Autodesk Inventor part; units mm, degrees
(part 2 of 3)
  arc A210 (-114.4847, -238.4545) -> (-108.2711, -237.6145) centre (-111.4451, -237.537) ccw projected
  arc A211 (-82.9809, -239.5618) -> (-81.2537, -236.3199) centre (-93.2079, -232.032) ccw projected
  arc A212 (-79.039, -235.4413) -> (-81.2537, -236.3199) centre (-79.7594, -236.8559) ccw projected
  line L73 (-79.039, -235.4413) -> (-73.2785, -238.3744) projected
  arc A213 (-72.5842, -240.5094) -> (-73.2785, -238.3744) centre (-73.9989, -239.7891) ccw projected
  line L74 (-72.5842, -240.5094) -> (-73.4026, -242.1166) projected
  arc A214 (-82.2866, -251.3886) -> (-73.4026, -242.1166) centre (-93.2079, -232.032) ccw projected
  arc A215 (-86.1924, -246.4835) -> (-82.2866, -251.3886) centre (-83.8468, -248.6233) ccw projected
  arc A216 (-86.1924, -246.4835) -> (-82.9809, -239.5618) centre (-95.5749, -237.9244) ccw projected
  line L75 (-36.7385, 25.1704) -> (-35.059, 27.3253) projected
  arc A217 (-31.1029, 31.7555) -> (-35.059, 27.3253) centre (0, 0) ccw projected
  arc A218 (-25.7245, 29.1468) -> (-31.1029, 31.7555) centre (-28.8812, 29.4873) ccw projected
  arc A219 (-25.7245, 29.1468) -> (-25.6629, 24.5535) centre (-6.7844, 27.1038) ccw projected
  arc A220 (-28.6757, 20.9563) -> (-25.6629, 24.5535) centre (-28.8093, 24.1285) ccw projected
  arc A221 (-28.6757, 20.9563) -> (-33.3257, 20.1764) centre (-27.8737, 1.9232) ccw projected
  arc A222 (-36.7385, 25.1704) -> (-33.3257, 20.1764) centre (-34.2343, 23.2186) ccw projected
  arc A223 (35.5169, -0.0989) -> (38.7459, 3.1685) centre (23.6807, 14.8279) ccw projected
  arc A224 (44.4304, 1.3195) -> (38.7459, 3.1685) centre (41.2568, 1.2252) ccw projected
  arc A225 (43.8282, -7.409) -> (44.4304, 1.3195) centre (0, 0) ccw projected
  arc A226 (37.9436, -8.4597) -> (43.8282, -7.409) centre (40.6976, -6.8798) ccw projected
  arc A227 (37.9436, -8.4597) -> (35.1939, -4.7799) centre (21.4199, -17.9397) ccw projected
  arc A228 (35.5169, -0.0989) -> (35.1939, -4.7799) centre (37.4896, -2.5866) ccw projected
  arc A229 (11.0693, 33.748) -> (8.9598, 37.8287) centre (-6.7844, 27.1038) ccw projected
  arc A230 (12.4749, 42.6636) -> (8.9598, 37.8287) centre (11.5838, 39.6162) ccw projected
  arc A231 (20.59, 39.3936) -> (12.4749, 42.6636) centre (0, 0) ccw projected
  arc A232 (19.7709, 33.4723) -> (20.59, 39.3936) centre (19.1193, 36.5798) ccw projected
  arc A233 (19.7709, 33.4723) -> (15.4215, 31.9943) centre (23.6807, 14.8279) ccw projected
  arc A234 (11.0693, 33.748) -> (15.4215, 31.9943) centre (14.045, 34.8554) ccw projected
  point P0 (0, 0)
  point P1 (-30.4878, -157.8365)
  point P2 (-86.8989, -84.1298)
  point P3 (-18.5783, -126.792)
  point P4 (-86.8983, -84.1302)
  point P5 (-76.7727, -34.3493)
  point P6 (-67.7312, -21.3007)
  point P7 (0, 0)
  point P8 (-18.8807, -57.2232)
  point P9 (-82.9011, -196.1535)
  point P10 (-20.9933, -42.0397)
  point P11 (0.0004, -0.0002)
  constraints: 15 other
extrude "Extrusion5" cut sketch "Sketch5" against normal blind 6.35 contours A22 A21 | A24 A23 | A26 A25 | A28 A27 | A30 A29
sketch "Sketch6" plane through (0, 0, 0) normal (0, 0, -1) x (-1, 0, 0)
  arc A0 (101.2304, -186.356) -> (103.5999, -188.8102) centre (104.3416, -185.7231) ccw projected
  arc A1 (110.0732, -190.9008) -> (103.5999, -188.8102) centre (93.216, -232.0303) ccw projected
  arc A2 (110.0732, -190.9008) -> (114.3886, -187.3301) centre (111.2773, -187.963) ccw projected
  line L0 (114.3886, -187.3301) -> (83.0114, -33.0802) projected
  arc A3 (83.0114, -33.0802) -> (70.7659, -6.3845) centre (19.7244, -45.9539) ccw projected
  arc A4 (70.7659, -6.3845) -> (65.1453, -8.9627) centre (68.2566, -8.3298) ccw projected
  line L1 (65.1453, -8.9627) -> (101.2304, -186.356) projected
  circle A5 centre (97.0428, -133.914) radius 2.413 projected
  circle A6 centre (86.9165, -84.1335) radius 2.413 projected
  circle A7 centre (107.169, -183.6945) radius 2.413 projected
  circle A8 centre (76.7902, -34.353) radius 2.413 projected
  point P0 (0, 0)
extrude "Extrusion6" cut sketch "Sketch6" against normal blind 6.35 contours A5 | A6 | A7 | A8
chamfer "Chamfer3" distance 3.175 angle 45 4 edges at (-74.3772, -34.353, 6.35) (-84.5035, -84.1335, 6.35) (-94.6298, -133.914, 6.35) (-104.756, -183.6945, 6.35)
sketch "Sketch7" plane through (0, 0, 6.35) normal (0, 0, 1) x (1, 0, 0)
  circle A0 centre (12.3653, -76.0452) radius 2.413 projected
  circle A1 centre (-52.177, -202.7989) radius 2.413 projected
  circle A2 centre (-19.9058, -139.422) radius 2.413 projected
  arc A3 (21.5354, -72.0292) -> (17.8927, -67.5194) centre (18.706, -70.5885) ccw projected
  line L0 (-48.8239, -210.2069) -> (21.5354, -72.0292) projected
  arc A4 (-54.4236, -210.3173) -> (-48.8239, -210.2069) centre (-51.6533, -208.7662) ccw projected
  arc A5 (-54.4236, -210.3173) -> (-58.1907, -204.654) centre (-93.2088, -232.0316) ccw projected
  arc A6 (-58.5187, -201.2578) -> (-58.1907, -204.654) centre (-55.6894, -202.6984) ccw projected
  line L1 (7.9149, -70.7896) -> (-58.5187, -201.2578) projected
  arc A7 (10.2771, -69.0898) -> (7.9149, -70.7896) centre (10.7442, -72.2303) ccw projected
  arc A8 (10.2771, -69.0898) -> (17.8927, -67.5194) centre (0, 0) ccw projected
  point P0 (0, 0)
extrude "Extrusion7" cut sketch "Sketch7" against normal blind 6.35 contours A0 | A1 | A2
chamfer "Chamfer4" distance 3.175 angle 45 3 edges at (9.9523, -76.0452, 6.35) (-22.3188, -139.422, 6.35) (-54.59, -202.7989, 6.35)
sketch "Sketch8" plane through (0, 0, 6.35) normal (0, 0, 1) x (1, 0, 0)
  line L0 (-60.6625, -189.7642) -> (-88.5389, -146.9454) projected
  arc A0 (-88.5389, -146.9454) -> (-92.3649, -145.7242) centre (-91.1997, -148.6777) ccw projected
  arc A1 (-96.1327, -146.5788) -> (-92.3649, -145.7242) centre (-97.0253, -133.9102) ccw projected
  arc A2 (-96.1327, -146.5788) -> (-99.0208, -149.1131) centre (-95.9095, -149.746) ccw projected
  line L1 (-99.0208, -149.1131) -> (-103.0492, -168.9165) projected
  arc A3 (-103.0492, -168.9165) -> (-101.3806, -172.3776) centre (-99.9379, -169.5493) ccw projected
  arc A4 (-94.5445, -182.1568) -> (-101.3806, -172.3776) centre (-107.1516, -183.6907) ccw projected
  arc A5 (-94.5445, -182.1568) -> (-92.4352, -184.7723) centre (-91.3928, -181.7733) ccw projected
  line L2 (-92.4352, -184.7723) -> (-64.3907, -194.5202) projected
  arc A6 (-64.3907, -194.5202) -> (-61.1139, -193.7769) centre (-63.3483, -191.5212) ccw projected
  arc A7 (-61.0938, -193.7571) -> (-61.1139, -193.7769) centre (-52.1761, -202.7994) ccw projected
  arc A8 (-61.0938, -193.7571) -> (-60.6625, -189.7642) centre (-63.3233, -191.4965) ccw projected
  line L3 (-39.1874, -128.4482) -> (-78.3296, -96.1425) projected
  arc A9 (-86.0064, -96.7983) -> (-81.6603, -95.6989) centre (-86.899, -84.1297) ccw projected
  arc A10 (-86.0064, -96.7983) -> (-88.8946, -99.3326) centre (-85.7833, -99.9655) ccw projected
  line L4 (-88.8946, -99.3326) -> (-92.9229, -119.1359) projected
  arc A11 (-92.9229, -119.1359) -> (-91.2544, -122.5971) centre (-89.8116, -119.7688) ccw projected
  arc A12 (-85.2514, -129.1495) -> (-91.2544, -122.5971) centre (-97.0253, -133.9102) ccw projected
  arc A13 (-85.2514, -129.1495) -> (-82.5342, -131.1262) centre (-82.3079, -127.9593) ccw projected
  line L5 (-82.5342, -131.1262) -> (-51.9243, -133.3141) projected
  arc A14 (-49.8924, -133.4593) -> (-51.9243, -133.3141) centre (-51.8109, -146.0136) ccw projected
  line L6 (-49.8924, -133.4593) -> (-41.4348, -134.0638) projected
  arc A15 (-41.4348, -134.0638) -> (-39.1874, -128.4482) centre (-41.2084, -130.8969) ccw projected
  line L7 (-34.3965, -142.2063) -> (-35.7266, -142.1112) projected
  arc A16 (-35.7266, -142.1112) -> (-39.1245, -145.4252) centre (-35.9529, -145.2781) ccw projected
  arc A17 (-46.8252, -157.694) -> (-39.1245, -145.4252) centre (-51.8109, -146.0136) ccw projected
  line L8 (-46.8252, -157.694) -> (-63.3439, -164.7448) projected
  arc A18 (-63.3886, -164.7638) -> (-63.3439, -164.7448) centre (-68.3295, -153.0643) ccw projected
  arc A19 (-63.3886, -164.7638) -> (-64.8141, -169.4209) centre (-62.1533, -167.6886) ccw projected
  line L9 (-64.8141, -169.4209) -> (-52.1408, -188.8873) projected
  arc A20 (-52.1408, -188.8873) -> (-50.0192, -190.2839) centre (-49.48, -187.1551) ccw projected
  arc A21 (-49.6538, -190.3524) -> (-50.0192, -190.2839) centre (-52.1761, -202.7994) ccw projected
  arc A22 (-49.6538, -190.3524) -> (-46.1939, -188.6813) centre (-49.0232, -187.2407) ccw projected
  line L10 (-46.1939, -188.6813) -> (-27.8038, -152.5648) projected
  arc A23 (-27.8038, -152.5648) -> (-28.4876, -148.7838) centre (-30.6331, -151.1242) ccw projected
  arc A24 (-31.6794, -144.183) -> (-28.4876, -148.7838) centre (-19.9055, -139.4223) ccw projected
  arc A25 (-31.6794, -144.183) -> (-34.3965, -142.2063) centre (-34.6229, -145.3732) ccw projected
  circle A26 centre (-19.9055, -139.4223) radius 5.588 projected
  circle A27 centre (12.3652, -76.0452) radius 5.588 projected
  circle A28 centre (-52.1761, -202.7994) radius 5.588 projected
  circle A29 centre (-10.4425, -25.9152) radius 6.731 projected
  circle A30 centre (-6.7844, 27.1038) radius 6.731 projected
  line L11 (-56.4266, -250.7606) -> (56.5866, -28.8133) projected
  arc A31 (-133.6545, -223.8044) -> (-56.4266, -250.7606) centre (-93.2079, -232.032) ccw projected
  line L12 (-94.387, -30.7661) -> (-133.6545, -223.8044) projected
  arc A32 (-79.8174, 0.8878) -> (-94.387, -30.7661) centre (-19.7163, -45.9555) ccw projected
  line L13 (-50.0843, 39.0361) -> (-79.8174, 0.8878) projected
  arc A33 (56.5866, -28.8133) -> (-50.0843, 39.0361) centre (0, 0) ccw projected
  circle A34 centre (0, 0) radius 13.4938 projected
  line L14 (-92.6287, -239.1078) -> (-87.8947, -227.3231) projected
  arc A35 (-87.8947, -227.3231) -> (-93.7871, -224.9561) centre (-90.8409, -226.1396) ccw projected
  line L15 (-93.7871, -224.9561) -> (-98.521, -236.7409) projected
  arc A36 (-98.521, -236.7409) -> (-92.6287, -239.1078) centre (-95.5749, -237.9244) ccw projected
  circle A37 centre (23.6807, 14.8279) radius 6.731 projected
  circle A38 centre (-27.8737, 1.9232) radius 6.731 projected
  circle A39 centre (21.4199, -17.9397) radius 6.731 projected
  arc A40 (-106.259, -196.3593) -> (-98.2138, -192.7133) centre (-107.1516, -183.6907) ccw projected
  arc A41 (-106.259, -196.3593) -> (-109.1471, -198.8936) centre (-106.0358, -199.5265) ccw projected
  line L16 (-109.1471, -198.8936) -> (-109.9237, -202.7115) projected
  arc A42 (-109.9237, -202.7115) -> (-105.452, -206.2132) centre (-106.8124, -203.3444) ccw projected
  arc A43 (-67.5567, -219.4404) -> (-76.984, -208.5093) centre (-93.2079, -232.032) ccw projected
  arc A44 (-67.5567, -219.4404) -> (-61.8773, -219.482) centre (-64.7066, -218.0413) ccw projected
  line L17 (-61.8773, -219.482) -> (-60.0746, -215.9418) projected
  arc A45 (-60.0746, -215.9418) -> (-60.7584, -212.1608) centre (-62.9039, -214.5011) ccw projected
  arc A46 (-64.7831, -204.3333) -> (-60.7584, -212.1608) centre (-52.1761, -202.7994) ccw projected
  arc A47 (-64.7831, -204.3333) -> (-66.8925, -201.7178) centre (-67.9349, -204.7168) ccw projected
  line L18 (-66.8925, -201.7178) -> (-72.8356, -199.6521) projected
  arc A48 (-94.937, -191.9699) -> (-98.2138, -192.7133) centre (-95.9794, -194.9689) ccw projected
  line L19 (-62.2456, -36.9383) -> (-28.8339, -52.5673) projected
  arc A49 (1.0666, -66.5539) -> (4.4026, -66.1514) centre (2.4119, -63.6779) ccw projected
  arc A50 (14.8879, -63.5983) -> (4.4026, -66.1514) centre (12.3652, -76.0452) ccw projected
  arc A51 (14.8879, -63.5983) -> (18.348, -61.9272) centre (15.5186, -60.4865) ccw projected
  line L20 (18.348, -61.9272) -> (26.6735, -45.5766) projected
  arc A52 (26.6735, -45.5766) -> (22.335, -41.3425) centre (23.8442, -44.136) ccw projected
  arc A53 (-11.2736, -45.6176) -> (22.335, -41.3425) centre (0, 0) ccw projected
  arc A54 (-46.9122, 2.703) -> (-52.5861, 4.8375) centre (-50.0819, 2.8857) ccw projected
  line L21 (-52.5861, 4.8375) -> (-64.7921, -10.8231) projected
  arc A55 (-64.7921, -10.8231) -> (-70.5556, -19.8503) centre (-19.7163, -45.9555) ccw projected
  arc A56 (-70.5556, -19.8503) -> (-69.5395, -23.9103) centre (-67.7312, -21.3006) ccw projected
  arc A57 (-64.0748, -34.1198) -> (-69.5395, -23.9103) centre (-76.7728, -34.3492) ccw projected
  arc A58 (-64.0748, -34.1198) -> (-62.2456, -36.9383) centre (-60.9004, -34.0624) ccw projected
  arc A59 (-75.8802, -47.0178) -> (-68.8102, -44.243) centre (-76.7728, -34.3492) ccw projected
  arc A60 (-75.8802, -47.0178) -> (-78.7683, -49.5521) centre (-75.657, -50.185) ccw projected
  line L22 (-78.7683, -49.5521) -> (-82.7967, -69.3554) projected
  arc A61 (-82.7967, -69.3554) -> (-81.1281, -72.8166) centre (-79.6854, -69.9883) ccw projected
  arc A62 (-75.9857, -77.6344) -> (-81.1281, -72.8166) centre (-86.899, -84.1297) ccw projected
  arc A63 (-75.9857, -77.6344) -> (-72.9996, -79.1751) centre (-73.2574, -76.0105) ccw projected
  line L23 (-72.9996, -79.1751) -> (-14.1782, -74.3844) projected
  arc A64 (-14.1782, -74.3844) -> (-13.0907, -68.3439) centre (-14.436, -71.2199) ccw projected
  line L24 (-13.0907, -68.3439) -> (-65.4743, -43.8405) projected
  arc A65 (-65.4743, -43.8405) -> (-68.8102, -44.243) centre (-66.8195, -46.7164) ccw projected
  arc A66 (-17.3829, -126.9753) -> (-25.1442, -127.8531) centre (-19.9055, -139.4223) ccw projected
  arc A67 (-17.3829, -126.9753) -> (-13.923, -125.3043) centre (-16.7523, -123.8636) ccw projected
  line L25 (-13.923, -125.3043) -> (4.4671, -89.1879) projected
  arc A68 (4.4671, -89.1879) -> (3.7832, -85.4068) centre (1.6378, -87.7473) ccw projected
  arc A69 (1.4518, -82.5405) -> (3.7832, -85.4068) centre (12.3652, -76.0452) ccw projected
  arc A70 (1.4518, -82.5405) -> (-1.5342, -80.9998) centre (-1.2765, -84.1643) ccw projected
  line L26 (-1.5342, -80.9998) -> (-69.4404, -86.5304) projected
  arc A71 (-69.4404, -86.5304) -> (-71.2037, -92.1436) centre (-69.1827, -89.6949) ccw projected
  line L27 (-71.2037, -92.1436) -> (-28.4749, -127.4095) projected
  arc A72 (-28.4749, -127.4095) -> (-25.1442, -127.8531) centre (-26.4539, -124.9608) ccw projected
  circle A73 centre (-68.3295, -153.0643) radius 6.731 projected
  circle A74 centre (-51.8109, -146.0136) radius 6.731 projected
  line L28 (-76.8242, -201.4676) -> (-78.1275, -204.7122) projected
  line L29 (-16.1603, -58.4956) -> (1.0666, -66.5539) projected
  line L30 (-14.9815, -47.5164) -> (-17.7613, -54.4362) projected
  line L31 (-85.1984, -201.8718) -> (-84.1423, -199.2428) projected
  line L32 (-86.0461, -195.0603) -> (-94.937, -191.9699) projected
  arc A75 (-88.6509, -203.8227) -> (-105.452, -206.2132) centre (-93.2079, -232.032) ccw projected
  line L33 (-24.5425, -50.8749) -> (-22.0524, -44.676) projected
  arc A76 (-46.9122, 2.703) -> (-23.4164, -40.7398) centre (0, 0) ccw projected
  arc A77 (-72.8356, -199.6521) -> (-76.8242, -201.4676) centre (-73.878, -202.6511) ccw projected
  arc A78 (-78.1275, -204.7122) -> (-76.984, -208.5093) centre (-75.1814, -205.8957) ccw projected
  arc A79 (-11.2736, -45.6176) -> (-14.9815, -47.5164) centre (-12.0354, -48.6999) ccw projected
  arc A80 (-17.7613, -54.4362) -> (-16.1603, -58.4956) centre (-14.8151, -55.6197) ccw projected
  arc A81 (-78.3296, -96.1425) -> (-81.6603, -95.6989) centre (-80.3506, -98.5912) ccw projected
  arc A82 (-84.1423, -199.2428) -> (-86.0461, -195.0603) centre (-87.0885, -198.0593) ccw projected
  arc A83 (-88.6509, -203.8227) -> (-85.1984, -201.8718) centre (-88.1445, -200.6883) ccw projected
  arc A84 (-22.0524, -44.676) -> (-23.4164, -40.7398) centre (-24.9986, -43.4925) ccw projected
  arc A85 (-28.8339, -52.5673) -> (-24.5425, -50.8749) centre (-27.4887, -49.6914) ccw projected
  arc A86 (-82.2866, -251.3886) -> (-73.4026, -242.1166) centre (-93.2079, -232.032) ccw projected
  line L34 (-73.4026, -242.1166) -> (-72.5842, -240.5094) projected
  arc A87 (-72.5842, -240.5094) -> (-73.2785, -238.3744) centre (-73.9989, -239.7891) ccw projected
  line L35 (-73.2785, -238.3744) -> (-79.039, -235.4413) projected
  arc A88 (-79.039, -235.4413) -> (-81.2537, -236.3199) centre (-79.7594, -236.8559) ccw projected
  arc A89 (-82.9809, -239.5618) -> (-81.2537, -236.3199) centre (-93.2079, -232.032) ccw projected
  arc A90 (-86.1924, -246.4835) -> (-82.9809, -239.5618) centre (-95.5749, -237.9244) ccw projected
  arc A91 (-86.1924, -246.4835) -> (-82.2866, -251.3886) centre (-83.8468, -248.6233) ccw projected
  arc A92 (-107.2952, -233.0332) -> (-109.5924, -228.6991) centre (-110.2253, -231.8104) ccw projected
  line L36 (-109.5924, -228.6991) -> (-113.3713, -227.9304) projected
  arc A93 (-113.3713, -227.9304) -> (-115.2631, -229.2902) centre (-113.6877, -229.486) ccw projected
  arc A94 (-115.2631, -229.2902) -> (-114.4847, -238.4545) centre (-93.2079, -232.032) ccw projected
  arc A95 (-114.4847, -238.4545) -> (-108.2711, -237.6145) centre (-111.4451, -237.537) ccw projected
  arc A96 (-107.2952, -233.0332) -> (-108.2711, -237.6145) centre (-95.5749, -237.9244) ccw projected
  arc A97 (35.5169, -0.0989) -> (38.7459, 3.1685) centre (23.6807, 14.8279) ccw projected
  arc A98 (35.5169, -0.0989) -> (35.1939, -4.7799) centre (37.4896, -2.5866) ccw projected
  arc A99 (37.9436, -8.4597) -> (35.1939, -4.7799) centre (21.4199, -17.9397) ccw projected
  arc A100 (37.9436, -8.4597) -> (43.8282, -7.409) centre (40.6976, -6.8798) ccw projected
  arc A101 (43.8282, -7.409) -> (44.4304, 1.3195) centre (0, 0) ccw projected
  arc A102 (44.4304, 1.3195) -> (38.7459, 3.1685) centre (41.2568, 1.2252) ccw projected
  arc A103 (11.0693, 33.748) -> (8.9598, 37.8287) centre (-6.7844, 27.1038) ccw projected
  arc A104 (11.0693, 33.748) -> (15.4215, 31.9943) centre (14.045, 34.8554) ccw projected
  arc A105 (19.7709, 33.4723) -> (15.4215, 31.9943) centre (23.6807, 14.8279) ccw projected
  arc A106 (19.7709, 33.4723) -> (20.59, 39.3936) centre (19.1193, 36.5798) ccw projected
  arc A107 (20.59, 39.3936) -> (12.4749, 42.6636) centre (0, 0) ccw projected
  arc A108 (12.4749, 42.6636) -> (8.9598, 37.8287) centre (11.5838, 39.6162) ccw projected
  arc A109 (-31.1029, 31.7555) -> (-35.059, 27.3253) centre (0, 0) ccw projected
  line L37 (-35.059, 27.3253) -> (-36.7385, 25.1704) projected
  arc A110 (-36.7385, 25.1704) -> (-33.3257, 20.1764) centre (-34.2343, 23.2186) ccw projected
  arc A111 (-28.6757, 20.9563) -> (-33.3257, 20.1764) centre (-27.8737, 1.9232) ccw projected
  arc A112 (-28.6757, 20.9563) -> (-25.6629, 24.5535) centre (-28.8093, 24.1285) ccw projected
  arc A113 (-25.7245, 29.1468) -> (-25.6629, 24.5535) centre (-6.7844, 27.1038) ccw projected
  arc A114 (-25.7245, 29.1468) -> (-31.1029, 31.7555) centre (-28.8812, 29.4873) ccw projected
  point P0 (0, 0)
  point P1 (-93.2076, -232.0321)
  point P2 (0, 0)
extrude "Extrusion8" cut sketch "Sketch8" against normal blind 6.35 contours A8 A7 A6 L2 A5 A4 A3 L1 A2 A1 A0 L0 | A40 A48 L32 A82 L31 A83 A75 A42 L16 A41 | A43 A78 L28 A77 L18 A47 A46 A45 L17 A44 | A58 A57 A56 A55 L21 A54 A76 A84 L33 A85 L19 | L29 A80 L30 A79 A53 A52 L20 A51 A50 A49 | A59 A65 L24 A64 L23 A63 A62 A61 L22 A60 | A66 A72 L27 A71 L26 A70 A69 A68 L25 A67
sketch "Sketch9" plane through (0, 0, 6.35) normal (0, 0, 1) x (1, 0, 0)
  arc A0 (-88.6509, -203.8227) -> (-105.452, -206.2132) centre (-93.2079, -232.032) ccw projected
  arc A1 (-109.9237, -202.7115) -> (-105.452, -206.2132) centre (-106.8124, -203.3444) ccw projected
  line L0 (-109.9237, -202.7115) -> (-109.1471, -198.8936) projected
  arc A2 (-106.259, -196.3593) -> (-109.1471, -198.8936) centre (-106.0358, -199.5265) ccw projected
  arc A3 (-106.259, -196.3593) -> (-98.2138, -192.7133) centre (-107.1516, -183.6907) ccw projected
  arc A4 (-94.937, -191.9699) -> (-98.2138, -192.7133) centre (-95.9794, -194.9689) ccw projected
  line L1 (-94.937, -191.9699) -> (-86.0461, -195.0603) projected
  arc A5 (-84.1423, -199.2428) -> (-86.0461, -195.0603) centre (-87.0885, -198.0593) ccw projected
  line L2 (-84.1423, -199.2428) -> (-85.1984, -201.8718) projected
  arc A6 (-88.6509, -203.8227) -> (-85.1984, -201.8718) centre (-88.1445, -200.6883) ccw projected
  arc A7 (-28.8339, -52.5673) -> (-24.5425, -50.8749) centre (-27.4887, -49.6914) ccw projected
  line L3 (-28.8339, -52.5673) -> (-62.2456, -36.9383) projected
  arc A8 (-64.0748, -34.1198) -> (-62.2456, -36.9383) centre (-60.9004, -34.0624) ccw projected
  arc A9 (-64.0748, -34.1198) -> (-69.5395, -23.9103) centre (-76.7728, -34.3492) ccw projected
  arc A10 (-70.5556, -19.8503) -> (-69.5395, -23.9103) centre (-67.7312, -21.3006) ccw projected
  arc A11 (-64.7921, -10.8231) -> (-70.5556, -19.8503) centre (-19.7163, -45.9555) ccw projected
  line L4 (-64.7921, -10.8231) -> (-52.5861, 4.8375) projected
  arc A12 (-46.9122, 2.703) -> (-52.5861, 4.8375) centre (-50.0819, 2.8857) ccw projected
  arc A13 (-46.9122, 2.703) -> (-23.4164, -40.7398) centre (0, 0) ccw projected
  arc A14 (-22.0524, -44.676) -> (-23.4164, -40.7398) centre (-24.9986, -43.4925) ccw projected
  line L5 (-22.0524, -44.676) -> (-24.5425, -50.8749) projected
  arc A15 (-88.5389, -146.9454) -> (-92.3649, -145.7242) centre (-91.1997, -148.6777) ccw projected
  line L6 (-88.5389, -146.9454) -> (-60.6625, -189.7642) projected
  arc A16 (-61.0938, -193.7571) -> (-60.6625, -189.7642) centre (-63.3233, -191.4965) ccw projected
  arc A17 (-61.0938, -193.7571) -> (-61.1139, -193.7769) centre (-52.1761, -202.7994) ccw projected
  arc A18 (-64.3907, -194.5202) -> (-61.1139, -193.7769) centre (-63.3483, -191.5212) ccw projected
  line L7 (-64.3907, -194.5202) -> (-92.4352, -184.7723) projected
  arc A19 (-94.5445, -182.1568) -> (-92.4352, -184.7723) centre (-91.3928, -181.7733) ccw projected
  arc A20 (-94.5445, -182.1568) -> (-101.3806, -172.3776) centre (-107.1516, -183.6907) ccw projected
  arc A21 (-103.0492, -168.9165) -> (-101.3806, -172.3776) centre (-99.9379, -169.5493) ccw projected
  line L8 (-103.0492, -168.9165) -> (-99.0208, -149.1131) projected
  arc A22 (-96.1327, -146.5788) -> (-99.0208, -149.1131) centre (-95.9095, -149.746) ccw projected
  arc A23 (-96.1327, -146.5788) -> (-92.3649, -145.7242) centre (-97.0253, -133.9102) ccw projected
  arc A24 (-17.7613, -54.4362) -> (-16.1603, -58.4956) centre (-14.8151, -55.6197) ccw projected
  line L9 (-17.7613, -54.4362) -> (-14.9815, -47.5164) projected
  arc A25 (-11.2736, -45.6176) -> (-14.9815, -47.5164) centre (-12.0354, -48.6999) ccw projected
  arc A26 (-11.2736, -45.6176) -> (22.335, -41.3425) centre (0, 0) ccw projected
  arc A27 (26.6735, -45.5766) -> (22.335, -41.3425) centre (23.8442, -44.136) ccw projected
  line L10 (26.6735, -45.5766) -> (18.348, -61.9272) projected
  arc A28 (14.8879, -63.5983) -> (18.348, -61.9272) centre (15.5186, -60.4865) ccw projected
  arc A29 (14.8879, -63.5983) -> (4.4026, -66.1514) centre (12.3652, -76.0452) ccw projected
  arc A30 (1.0666, -66.5539) -> (4.4026, -66.1514) centre (2.4119, -63.6779) ccw projected
  line L11 (1.0666, -66.5539) -> (-16.1603, -58.4956) projected
  arc A31 (-75.9857, -77.6344) -> (-81.1281, -72.8166) centre (-86.899, -84.1297) ccw projected
  arc A32 (-82.7967, -69.3554) -> (-81.1281, -72.8166) centre (-79.6854, -69.9883) ccw projected
  line L12 (-82.7967, -69.3554) -> (-78.7683, -49.5521) projected
  arc A33 (-75.8802, -47.0178) -> (-78.7683, -49.5521) centre (-75.657, -50.185) ccw projected
  arc A34 (-75.8802, -47.0178) -> (-68.8102, -44.243) centre (-76.7728, -34.3492) ccw projected
  arc A35 (-65.4743, -43.8405) -> (-68.8102, -44.243) centre (-66.8195, -46.7164) ccw projected
  line L13 (-65.4743, -43.8405) -> (-13.0907, -68.3439) projected
  arc A36 (-14.1782, -74.3844) -> (-13.0907, -68.3439) centre (-14.436, -71.2199) ccw projected
  line L14 (-14.1782, -74.3844) -> (-72.9996, -79.1751) projected
  arc A37 (-75.9857, -77.6344) -> (-72.9996, -79.1751) centre (-73.2574, -76.0105) ccw projected
  arc A38 (1.4518, -82.5405) -> (3.7832, -85.4068) centre (12.3652, -76.0452) ccw projected
  arc A39 (4.4671, -89.1879) -> (3.7832, -85.4068) centre (1.6378, -87.7473) ccw projected
  line L15 (4.4671, -89.1879) -> (-13.923, -125.3043) projected
  arc A40 (-17.3829, -126.9753) -> (-13.923, -125.3043) centre (-16.7523, -123.8636) ccw projected
  arc A41 (-17.3829, -126.9753) -> (-25.1442, -127.8531) centre (-19.9055, -139.4223) ccw projected
  arc A42 (-28.4749, -127.4095) -> (-25.1442, -127.8531) centre (-26.4539, -124.9608) ccw projected
  line L16 (-28.4749, -127.4095) -> (-71.2037, -92.1436) projected
  arc A43 (-69.4404, -86.5304) -> (-71.2037, -92.1436) centre (-69.1827, -89.6949) ccw projected
  line L17 (-69.4404, -86.5304) -> (-1.5342, -80.9998) projected
  arc A44 (1.4518, -82.5405) -> (-1.5342, -80.9998) centre (-1.2765, -84.1643) ccw projected
  arc A45 (-64.7831, -204.3333) -> (-60.7584, -212.1608) centre (-52.1761, -202.7994) ccw projected
  arc A46 (-60.0746, -215.9418) -> (-60.7584, -212.1608) centre (-62.9039, -214.5011) ccw projected
  line L18 (-60.0746, -215.9418) -> (-61.8773, -219.482) projected
  arc A47 (-67.5567, -219.4404) -> (-61.8773, -219.482) centre (-64.7066, -218.0413) ccw projected
  arc A48 (-67.5567, -219.4404) -> (-76.984, -208.5093) centre (-93.2079, -232.032) ccw projected
  arc A49 (-78.1275, -204.7122) -> (-76.984, -208.5093) centre (-75.1814, -205.8957) ccw projected
  line L19 (-78.1275, -204.7122) -> (-76.8242, -201.4676) projected
  arc A50 (-72.8356, -199.6521) -> (-76.8242, -201.4676) centre (-73.878, -202.6511) ccw projected
  line L20 (-72.8356, -199.6521) -> (-66.8925, -201.7178) projected
  arc A51 (-64.7831, -204.3333) -> (-66.8925, -201.7178) centre (-67.9349, -204.7168) ccw projected
  circle A52 centre (-19.9058, -139.422) radius 5.588 projected
  circle A53 centre (-107.169, -183.6945) radius 5.588 projected
  circle A54 centre (-86.9165, -84.1335) radius 5.588 projected
  circle A55 centre (-56.5448, -157.7983) radius 6.731 projected
  line L21 (-98.521, -236.7409) -> (-93.7871, -224.9561) projected
  arc A56 (-87.8947, -227.3231) -> (-93.7871, -224.9561) centre (-90.8409, -226.1396) ccw projected
  line L22 (-87.8947, -227.3231) -> (-92.6287, -239.1078) projected
  arc A57 (-98.521, -236.7409) -> (-92.6287, -239.1078) centre (-95.5749, -237.9244) ccw projected
  circle A58 centre (0, 0) radius 13.4938 projected
  arc A59 (56.5866, -28.8133) -> (-50.0843, 39.0361) centre (0, 0) ccw projected
  line L23 (-50.0843, 39.0361) -> (-79.8174, 0.8878) projected
  arc A60 (-79.8174, 0.8878) -> (-94.387, -30.7661) centre (-19.7163, -45.9555) ccw projected
  line L24 (-94.387, -30.7661) -> (-133.6545, -223.8044) projected
  arc A61 (-133.6545, -223.8044) -> (-56.4266, -250.7606) centre (-93.2079, -232.032) ccw projected
  line L25 (-56.4266, -250.7606) -> (56.5866, -28.8133) projected
  circle A62 centre (-63.5956, -141.2796) radius 6.731 projected
  arc A63 (-11.6072, -28.8689) -> (-9.2419, -22.976) centre (-10.4066, -25.9296) ccw projected
  arc A64 (-9.2419, -22.976) -> (-11.6072, -28.8689) centre (-10.4425, -25.9152) ccw projected
  arc A65 (26.3454, 16.5542) -> (20.9946, 13.1351) centre (23.6593, 14.8615) ccw projected
  arc A66 (20.9946, 13.1351) -> (26.3454, 16.5542) centre (23.6807, 14.8279) ccw projected
  arc A67 (23.8979, -19.9247) -> (18.9666, -15.9242) centre (21.4446, -17.9092) ccw projected
  arc A68 (18.9666, -15.9242) -> (23.8979, -19.9247) centre (21.4199, -17.9397) ccw projected
  arc A69 (-7.5477, 30.1857) -> (-6.0599, 24.0126) centre (-6.8231, 27.0945) ccw projected
  arc A70 (-6.0599, 24.0126) -> (-7.5477, 30.1857) centre (-6.7844, 27.1038) ccw projected
  arc A71 (-31.0394, 2.1661) -> (-24.7113, 1.6412) centre (-27.877, 1.8842) ccw projected
  arc A72 (-24.7113, 1.6412) -> (-31.0394, 2.1661) centre (-27.8737, 1.9232) ccw projected
  circle A73 centre (-76.7902, -34.353) radius 5.588 projected
  circle A74 centre (-97.0428, -133.914) radius 5.588 projected
  circle A75 centre (12.3653, -76.0452) radius 5.588 projected
  circle A76 centre (-52.177, -202.7989) radius 5.588 projected
  circle A77 centre (-56.5448, -157.7983) radius 3.175 projected
  circle A78 centre (-56.5448, -157.7983) radius 12.7
  circle A79 centre (-63.5956, -141.2796) radius 12.7
  line L26 (-68.2253, -162.7839) -> (-75.2761, -146.2652)
  line L27 (-51.9151, -136.294) -> (-44.8643, -152.8126)
  circle A80 centre (-19.9058, -139.422) radius 2.413 projected
  circle A81 centre (-97.0428, -133.914) radius 2.413 projected
  line L28 (-19.9058, -139.422) -> (-97.0428, -133.914)
  circle A82 centre (-52.177, -202.7989) radius 2.413 projected
  line L29 (-97.0428, -133.914) -> (-52.177, -202.7989)
  line L30 (-57.4695, -187.6855) -> (-85.346, -144.8667)
  arc A83 (-85.346, -144.8667) -> (-93.763, -142.18) centre (-91.1997, -148.6777) ccw
  arc A84 (-96.4005, -142.7782) -> (-93.763, -142.18) centre (-97.0253, -133.9102) ccw
  arc A85 (-96.4005, -142.7782) -> (-102.7544, -148.3536) centre (-95.9095, -149.746) ccw
  line L31 (-102.7544, -148.3536) -> (-106.7827, -168.157)
  arc A86 (-106.7827, -168.157) -> (-103.1119, -175.7716) centre (-99.9379, -169.5493) ccw
  arc A87 (-98.3266, -182.617) -> (-103.1119, -175.7716) centre (-107.1516, -183.6907) ccw
  arc A88 (-98.3266, -182.617) -> (-93.6861, -188.3711) centre (-91.3928, -181.7733) ccw
  line L32 (-93.6861, -188.3711) -> (-65.6416, -198.119)
  arc A89 (-65.6416, -198.119) -> (-58.4325, -196.4836) centre (-63.3483, -191.5212) ccw
  arc A90 (-58.4185, -196.4698) -> (-58.4325, -196.4836) centre (-52.1761, -202.7994) ccw
  arc A91 (-58.4185, -196.4698) -> (-57.4695, -187.6855) centre (-63.3233, -191.4965) ccw
  line L33 (-19.6626, -135.6197) -> (-104.4206, -129.5675)
  line L34 (-104.4206, -129.5675) -> (-55.3665, -204.883)
  line L35 (-20.2053, -143.2204) -> (-89.6649, -138.2605)
  line L36 (-89.6649, -138.2605) -> (-48.9813, -200.7243)
  arc A92 (39.6106, -20.1693) -> (-35.059, 27.3253) centre (0, 0) ccw
  line L37 (-35.059, 27.3253) -> (-64.7921, -10.8231)
  arc A93 (-64.7921, -10.8231) -> (-75.7193, -34.5635) centre (-19.7163, -45.9555) ccw
  line L38 (-75.7193, -34.5635) -> (-114.9869, -227.6018)
  arc A94 (-114.9869, -227.6018) -> (-73.4026, -242.1166) centre (-93.2079, -232.032) ccw
  line L39 (-73.4026, -242.1166) -> (39.6106, -20.1693)
  line L40 (-76.0542, -98.0205) -> (-33.3253, -133.2864)
  arc A95 (-33.3253, -133.2864) -> (-22.001, -134.7946) centre (-26.4539, -124.9608) ccw
  arc A96 (-18.8965, -134.4435) -> (-22.001, -134.7946) centre (-19.9055, -139.4223) ccw
  arc A97 (-18.8965, -134.4435) -> (-7.1326, -128.7619) centre (-16.7523, -123.8636) ccw
  line L41 (-7.1326, -128.7619) -> (11.2575, -92.6455)
  arc A98 (11.2575, -92.6455) -> (8.9324, -79.7898) centre (1.6378, -87.7473) ccw
  arc A99 (7.9998, -78.6433) -> (8.9324, -79.7898) centre (12.3652, -76.0452) ccw
  arc A100 (7.9998, -78.6433) -> (-2.1528, -73.405) centre (-1.2765, -84.1643) ccw
  line L42 (-2.1528, -73.405) -> (-70.059, -78.9356)
  arc A101 (-70.059, -78.9356) -> (-76.0542, -98.0205) centre (-69.1827, -89.6949) ccw
  spline S0 degree 4 poles (-63.6141, -178.2577) (-65.5437, -175.2953) (-66.9719, -169.1994) (-60.6632, -170.3495) (-57.0322, -170.4889) knots 0 0 0 0 0 1 1 1 1 1
  circle A102 centre (-52.177, -202.7989) radius 12.7002
  circle A103 centre (-56.5448, -157.7983) radius 3.175 projected
  spline S1 degree 1 poles (-56.5448, -157.7983) (-35.8374, -168.3422) knots 0 0 1 1
  circle A104 centre (-19.9058, -139.422) radius 12.6998
  spline S2 degree 3 poles (-54.816, -154.4031) (-47.9136, -157.9177) (-41.0111, -161.4324) (-34.1086, -164.9471) knots 0 0 0 0 1 1 1 1
  spline S3 degree 3 poles (-58.2736, -161.1935) (-51.3712, -164.7081) (-44.4687, -168.2228) (-37.5662, -171.7374) knots 0 0 0 0 1 1 1 1
  point P0 (0, 0)
  point P1 (-64.3387, -171.811)
  point P2 (-47.4776, -166.6907)
  point P3 (-55.5965, -190.5677)
  point P4 (-47.3921, -191.0345)
  point P5 (-26.6052, -150.211)
  point P6 (-32.2612, -142.3595)
  point P7 (-49.8626, -141.1026)
  point P8 (-44.02, -159.9003)
  point P9 (-34.108, -164.9472)
  dimension "d37" = 3.81
  dimension "d38" = 3.81
  dimension "d30" = 25.4
  dimension "d31" = 25.4
  dimension "d32" = 3.81
  dimension "d33" = 3.81
  dimension "d34" = 3.81
  dimension "d35" = 19.05
  dimension "d36" = 7.62
  constraints: 43 point on circle, 34 end point, 23 centre point, 4 coincident, 3 point on line, 3 tangent, 1 parallel, 40 other
  measures "d30" diameter of A78
  measures "d31" diameter of A79
  measures "d32" distance between parallel lines of L6 L30
  measures "d33" distance between parallel lines of L28 L33
  measures "d34" distance between parallel lines of L28 L35
  measures "d35" distance between parallel lines of L25 L39
  measures "d36" distance between parallel lines of L16 L40
extrude "Extrusion9" [suppressed]
fillet "Fillet1" [suppressed]
sketch "Sketch10" plane through (0, 0, 6.35) normal (0, 0, 1) x (1, 0, 0)
  arc A0 (-88.6509, -203.8227) -> (-105.452, -206.2132) centre (-93.2079, -232.032) ccw projected
  arc A1 (-109.9237, -202.7115) -> (-105.452, -206.2132) centre (-106.8124, -203.3444) ccw projected
  line L0 (-109.9237, -202.7115) -> (-109.1471, -198.8936) projected
  arc A2 (-106.259, -196.3593) -> (-109.1471, -198.8936) centre (-106.0358, -199.5265) ccw projected
  arc A3 (-106.259, -196.3593) -> (-98.2138, -192.7133) centre (-107.1516, -183.6907) ccw projected
  arc A4 (-94.937, -191.9699) -> (-98.2138, -192.7133) centre (-95.9794, -194.9689) ccw projected
  line L1 (-94.937, -191.9699) -> (-86.0461, -195.0603) projected
  arc A5 (-84.1423, -199.2428) -> (-86.0461, -195.0603) centre (-87.0885, -198.0593) ccw projected
  line L2 (-84.1423, -199.2428) -> (-85.1984, -201.8718) projected
  arc A6 (-88.6509, -203.8227) -> (-85.1984, -201.8718) centre (-88.1445, -200.6883) ccw projected
  arc A7 (-28.8339, -52.5673) -> (-24.5425, -50.8749) centre (-27.4887, -49.6914) ccw projected
  line L3 (-28.8339, -52.5673) -> (-62.2456, -36.9383) projected
  arc A8 (-64.0748, -34.1198) -> (-62.2456, -36.9383) centre (-60.9004, -34.0624) ccw projected
  arc A9 (-64.0748, -34.1198) -> (-69.5395, -23.9103) centre (-76.7728, -34.3492) ccw projected
  arc A10 (-70.5556, -19.8503) -> (-69.5395, -23.9103) centre (-67.7312, -21.3006) ccw projected
  arc A11 (-64.7921, -10.8231) -> (-70.5556, -19.8503) centre (-19.7163, -45.9555) ccw projected
  line L4 (-64.7921, -10.8231) -> (-52.5861, 4.8375) projected
  arc A12 (-46.9122, 2.703) -> (-52.5861, 4.8375) centre (-50.0819, 2.8857) ccw projected
  arc A13 (-46.9122, 2.703) -> (-23.4164, -40.7398) centre (0, 0) ccw projected
  arc A14 (-22.0524, -44.676) -> (-23.4164, -40.7398) centre (-24.9986, -43.4925) ccw projected
  line L5 (-22.0524, -44.676) -> (-24.5425, -50.8749) projected
  arc A15 (-88.5389, -146.9454) -> (-92.3649, -145.7242) centre (-91.1997, -148.6777) ccw projected
  line L6 (-88.5389, -146.9454) -> (-60.6625, -189.7642) projected
  arc A16 (-61.0938, -193.7571) -> (-60.6625, -189.7642) centre (-63.3233, -191.4965) ccw projected
  arc A17 (-61.0938, -193.7571) -> (-61.1139, -193.7769) centre (-52.1761, -202.7994) ccw projected
  arc A18 (-64.3907, -194.5202) -> (-61.1139, -193.7769) centre (-63.3483, -191.5212) ccw projected
  line L7 (-64.3907, -194.5202) -> (-92.4352, -184.7723) projected
  arc A19 (-94.5445, -182.1568) -> (-92.4352, -184.7723) centre (-91.3928, -181.7733) ccw projected
  arc A20 (-94.5445, -182.1568) -> (-101.3806, -172.3776) centre (-107.1516, -183.6907) ccw projected
  arc A21 (-103.0492, -168.9165) -> (-101.3806, -172.3776) centre (-99.9379, -169.5493) ccw projected
  line L8 (-103.0492, -168.9165) -> (-99.0208, -149.1131) projected
  arc A22 (-96.1327, -146.5788) -> (-99.0208, -149.1131) centre (-95.9095, -149.746) ccw projected
  arc A23 (-96.1327, -146.5788) -> (-92.3649, -145.7242) centre (-97.0253, -133.9102) ccw projected
  arc A24 (-17.7613, -54.4362) -> (-16.1603, -58.4956) centre (-14.8151, -55.6197) ccw projected
  line L9 (-17.7613, -54.4362) -> (-14.9815, -47.5164) projected
  arc A25 (-11.2736, -45.6176) -> (-14.9815, -47.5164) centre (-12.0354, -48.6999) ccw projected
  arc A26 (-11.2736, -45.6176) -> (22.335, -41.3425) centre (0, 0) ccw projected
  arc A27 (26.6735, -45.5766) -> (22.335, -41.3425) centre (23.8442, -44.136) ccw projected
  line L10 (26.6735, -45.5766) -> (18.348, -61.9272) projected
  arc A28 (14.8879, -63.5983) -> (18.348, -61.9272) centre (15.5186, -60.4865) ccw projected
  arc A29 (14.8879, -63.5983) -> (4.4026, -66.1514) centre (12.3652, -76.0452) ccw projected
  arc A30 (1.0666, -66.5539) -> (4.4026, -66.1514) centre (2.4119, -63.6779) ccw projected
  line L11 (1.0666, -66.5539) -> (-16.1603, -58.4956) projected
  arc A31 (-75.9857, -77.6344) -> (-81.1281, -72.8166) centre (-86.899, -84.1297) ccw projected
  arc A32 (-82.7967, -69.3554) -> (-81.1281, -72.8166) centre (-79.6854, -69.9883) ccw projected
  line L12 (-82.7967, -69.3554) -> (-78.7683, -49.5521) projected
  arc A33 (-75.8802, -47.0178) -> (-78.7683, -49.5521) centre (-75.657, -50.185) ccw projected
  arc A34 (-75.8802, -47.0178) -> (-68.8102, -44.243) centre (-76.7728, -34.3492) ccw projected
  arc A35 (-65.4743, -43.8405) -> (-68.8102, -44.243) centre (-66.8195, -46.7164) ccw projected
  line L13 (-65.4743, -43.8405) -> (-13.0907, -68.3439) projected
  arc A36 (-14.1782, -74.3844) -> (-13.0907, -68.3439) centre (-14.436, -71.2199) ccw projected
  line L14 (-14.1782, -74.3844) -> (-72.9996, -79.1751) projected
  arc A37 (-75.9857, -77.6344) -> (-72.9996, -79.1751) centre (-73.2574, -76.0105) ccw projected
  arc A38 (1.4518, -82.5405) -> (3.7832, -85.4068) centre (12.3652, -76.0452) ccw projected
  arc A39 (4.4671, -89.1879) -> (3.7832, -85.4068) centre (1.6378, -87.7473) ccw projected
  line L15 (4.4671, -89.1879) -> (-13.923, -125.3043) projected
  arc A40 (-17.3829, -126.9753) -> (-13.923, -125.3043) centre (-16.7523, -123.8636) ccw projected
  arc A41 (-17.3829, -126.9753) -> (-25.1442, -127.8531) centre (-19.9055, -139.4223) ccw projected
  arc A42 (-28.4749, -127.4095) -> (-25.1442, -127.8531) centre (-26.4539, -124.9608) ccw projected
  line L16 (-28.4749, -127.4095) -> (-71.2037, -92.1436) projected
  arc A43 (-69.4404, -86.5304) -> (-71.2037, -92.1436) centre (-69.1827, -89.6949) ccw projected
  line L17 (-69.4404, -86.5304) -> (-1.5342, -80.9998) projected
  arc A44 (1.4518, -82.5405) -> (-1.5342, -80.9998) centre (-1.2765, -84.1643) ccw projected
  arc A45 (-64.7831, -204.3333) -> (-60.7584, -212.1608) centre (-52.1761, -202.7994) ccw projected
  arc A46 (-60.0746, -215.9418) -> (-60.7584, -212.1608) centre (-62.9039, -214.5011) ccw projected
  line L18 (-60.0746, -215.9418) -> (-61.8773, -219.482) projected
  arc A47 (-67.5567, -219.4404) -> (-61.8773, -219.482) centre (-64.7066, -218.0413) ccw projected
  arc A48 (-67.5567, -219.4404) -> (-76.984, -208.5093) centre (-93.2079, -232.032) ccw projected
  arc A49 (-78.1275, -204.7122) -> (-76.984, -208.5093) centre (-75.1814, -205.8957) ccw projected
  line L19 (-78.1275, -204.7122) -> (-76.8242, -201.4676) projected
  arc A50 (-72.8356, -199.6521) -> (-76.8242, -201.4676) centre (-73.878, -202.6511) ccw projected
  line L20 (-72.8356, -199.6521) -> (-66.8925, -201.7178) projected
  arc A51 (-64.7831, -204.3333) -> (-66.8925, -201.7178) centre (-67.9349, -204.7168) ccw projected
  circle A52 centre (-19.9058, -139.422) radius 5.588 projected
  circle A53 centre (-107.169, -183.6945) radius 5.588 projected
  circle A54 centre (-86.9165, -84.1335) radius 5.588 projected
  circle A55 centre (-56.5448, -157.7983) radius 6.731 projected
  line L21 (-98.521, -236.7409) -> (-93.7871, -224.9561) projected
  arc A56 (-87.8947, -227.3231) -> (-93.7871, -224.9561) centre (-90.8409, -226.1396) ccw projected
  line L22 (-87.8947, -227.3231) -> (-92.6287, -239.1078) projected
  arc A57 (-98.521, -236.7409) -> (-92.6287, -239.1078) centre (-95.5749, -237.9244) ccw projected
  circle A58 centre (0, 0) radius 13.4938 projected
  arc A59 (56.5866, -28.8133) -> (-50.0843, 39.0361) centre (0, 0) ccw projected
  line L23 (-50.0843, 39.0361) -> (-79.8174, 0.8878) projected
  arc A60 (-79.8174, 0.8878) -> (-94.387, -30.7661) centre (-19.7163, -45.9555) ccw projected
  line L24 (-94.387, -30.7661) -> (-133.6545, -223.8044) projected
  arc A61 (-133.6545, -223.8044) -> (-56.4266, -250.7606) centre (-93.2079, -232.032) ccw projected
  line L25 (-56.4266, -250.7606) -> (56.5866, -28.8133) projected
  circle A62 centre (-63.5956, -141.2796) radius 6.731 projected
  arc A63 (-11.6072, -28.8689) -> (-9.2419, -22.976) centre (-10.4066, -25.9296) ccw projected
  arc A64 (-9.2419, -22.976) -> (-11.6072, -28.8689) centre (-10.4425, -25.9152) ccw projected
  arc A65 (26.3454, 16.5542) -> (20.9946, 13.1351) centre (23.6593, 14.8615) ccw projected
  arc A66 (20.9946, 13.1351) -> (26.3454, 16.5542) centre (23.6807, 14.8279) ccw projected
  arc A67 (23.8979, -19.9247) -> (18.9666, -15.9242) centre (21.4446, -17.9092) ccw projected
  arc A68 (18.9666, -15.9242) -> (23.8979, -19.9247) centre (21.4199, -17.9397) ccw projected
  arc A69 (-7.5477, 30.1857) -> (-6.0599, 24.0126) centre (-6.8231, 27.0945) ccw projected
  arc A70 (-6.0599, 24.0126) -> (-7.5477, 30.1857) centre (-6.7844, 27.1038) ccw projected
  arc A71 (-31.0394, 2.1661) -> (-24.7113, 1.6412) centre (-27.877, 1.8842) ccw projected
  arc A72 (-24.7113, 1.6412) -> (-31.0394, 2.1661) centre (-27.8737, 1.9232) ccw projected
  circle A73 centre (-76.7902, -34.353) radius 5.588 projected
  circle A74 centre (-97.0428, -133.914) radius 5.588 projected
  circle A75 centre (12.3653, -76.0452) radius 5.588 projected
  circle A76 centre (-52.177, -202.7989) radius 5.588 projected
  line L26 (-76.0542, -98.0205) -> (-33.3253, -133.2864)
  arc A77 (-33.3253, -133.2864) -> (-22.001, -134.7946) centre (-26.4539, -124.9608) ccw
  arc A78 (-18.8965, -134.4435) -> (-22.001, -134.7946) centre (-19.9055, -139.4223) ccw
  arc A79 (-18.8965, -134.4435) -> (-7.1326, -128.7619) centre (-16.7523, -123.8636) ccw
  line L27 (-7.1326, -128.7619) -> (11.2575, -92.6455)
  arc A80 (11.2575, -92.6455) -> (8.9324, -79.7898) centre (1.6378, -87.7473) ccw
  arc A81 (7.9998, -78.6433) -> (8.9324, -79.7898) centre (12.3652, -76.0452) ccw
  arc A82 (7.9998, -78.6433) -> (-2.1528, -73.405) centre (-1.2765, -84.1643) ccw
  line L28 (-2.1528, -73.405) -> (-70.059, -78.9356)
  arc A83 (-70.059, -78.9356) -> (-76.0542, -98.0205) centre (-69.1827, -89.6949) ccw
  line L29 (-54.2766, -185.6068) -> (-82.153, -142.788)
  arc A84 (-82.153, -142.788) -> (-95.1611, -138.6358) centre (-91.1997, -148.6777) ccw
  arc A85 (-96.6683, -138.9777) -> (-95.1611, -138.6358) centre (-97.0253, -133.9102) ccw
  arc A86 (-96.6683, -138.9777) -> (-106.4879, -147.5941) centre (-95.9095, -149.746) ccw
  line L30 (-106.4879, -147.5941) -> (-110.5163, -167.3975)
  arc A87 (-110.5163, -167.3975) -> (-104.8432, -179.1655) centre (-99.9379, -169.5493) ccw
  arc A88 (-102.1088, -183.0772) -> (-104.8432, -179.1655) centre (-107.1516, -183.6907) ccw
  arc A89 (-102.1088, -183.0772) -> (-94.937, -191.9699) centre (-91.3928, -181.7733) ccw
  line L31 (-94.937, -191.9699) -> (-66.8925, -201.7178)
  arc A90 (-66.8925, -201.7178) -> (-55.7512, -199.1904) centre (-63.3483, -191.5212) ccw
  arc A91 (-55.7432, -199.1825) -> (-55.7512, -199.1904) centre (-52.1761, -202.7994) ccw
  arc A92 (-55.7432, -199.1825) -> (-54.2766, -185.6068) centre (-63.3233, -191.4965) ccw
  line L32 (-114.9869, -227.6018) -> (-75.7193, -34.5635)
  arc A93 (-64.7921, -10.8231) -> (-75.7193, -34.5635) centre (-19.7163, -45.9555) ccw
  line L33 (-64.7921, -10.8231) -> (-35.059, 27.3253)
  arc A94 (39.6106, -20.1693) -> (-35.059, 27.3253) centre (0, 0) ccw
  line L34 (39.6106, -20.1693) -> (-73.4026, -242.1166)
  arc A95 (-114.9869, -227.6018) -> (-73.4026, -242.1166) centre (-93.2079, -232.032) ccw
  circle A96 centre (-86.9165, -84.1335) radius 5.588 projected
  circle A97 centre (-86.9165, -84.1335) radius 12.6842
  circle A98 centre (-97.0428, -133.914) radius 12.729
  circle A99 centre (-63.5956, -141.2796) radius 12.7
  spline S0 degree 4 poles (-85.5845, -139.4581) (-82.6048, -141.2729) (-78.0759, -144.0098) (-76.3932, -137.6156) (-74.1963, -134.2857) knots 0 0 0 0 0 1 1 1 1 1
  line L35 (-33.8531, -134.6059) -> (-44.1315, -133.8713)
  arc A100 (-44.1315, -133.8713) -> (-54.8294, -148.8767) centre (-44.901, -144.6389) ccw
  line L36 (-54.8294, -148.8767) -> (-51.8726, -155.8039)
  arc A101 (-51.4654, -157.8762) -> (-51.8726, -155.8039) centre (-56.5448, -157.7982) ccw
  arc A102 (-51.4654, -157.8762) -> (-45.5699, -167.6619) centre (-40.6717, -158.0422) ccw
  line L37 (-45.5699, -167.6619) -> (-40.3955, -170.2966)
  arc A103 (-40.3955, -170.2966) -> (-25.8776, -165.5752) centre (-35.4973, -160.6769) ccw
  line L38 (-25.8776, -165.5752) -> (-21.0133, -156.0222)
  arc A104 (-21.0133, -156.0222) -> (-23.3382, -143.1667) centre (-30.633, -151.1239) ccw
  arc A105 (-24.6148, -141.3266) -> (-23.3382, -143.1667) centre (-19.9055, -139.4223) ccw
  arc A106 (-24.6148, -141.3266) -> (-33.8531, -134.6059) centre (-34.6226, -145.3734) ccw
  circle A107 centre (-36.3666, -132.8347) radius 1.5875
  point P0 (0, 0)
  point P1 (-79.4783, -141.0424)
  point P2 (-36.4798, -134.4181)
  point P3 (-35.3561, -131.6103)
  point P4 (-79.0465, -94.081)
  point P5 (-88.3661, -96.7346)
  point P6 (-93.4453, -121.7039)
  point P7 (-74.636, -135.0027)
  point P8 (-51.8719, -136.3964)
  dimension "d45" = 25.4
  dimension "d42" = 7.62
  dimension "d43" = 7.62
  dimension "d44" = 19.05
  dimension "d47" = 3.175
  constraints: 53 point on circle, 28 centre point, 26 end point, 3 coincident, 2 tangent, 35 other
  measures "d42" distance between parallel lines of L16 L26
  measures "d43" distance between parallel lines of L6 L29
  measures "d44" distance between parallel lines of L24 L32
  measures "d47" diameter of A107
extrude "Extrusion10" cut sketch "Sketch10" against normal blind 6.35 contours S0 A98 L32 A97 A83 L26 A107 L35 A100 A99 | A107